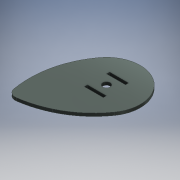
# Autodesk Inventor part: leva00
Saved by Autodesk Inventor 2016 (Build 200138000, 138)
## iProperties
Created: 2016-09-20
Part Number: leva00
Material: Madera (abedul)
Document SubType Name: Modeling
Designer: i95sa
Density: 0.55 g/cm^3
Appearance: Gris plomo - Pulido
Author: i95sa
Autodesk Inventor part; units mm, degrees
ref_plane "YZ Plane" through (0, 0, 0) normal (1, 0, 0) x (0, 1, 0)
ref_plane "XZ Plane" through (0, 0, 0) normal (0, 1, 0) x (-1, 0, 0)
ref_plane "XY Plane" through (0, 0, 0) normal (0, 0, 1) x (1, 0, 0)
sketch "Boceto1" plane through (0, 0, 0) normal (0, 0, 1) x (1, 0, 0)
  arc A0 (26.1711, 36.0215) -> (-26.1711, -36.0215) centre (0, 0) ccw
  arc A1 (-40.2753, -55.4342) -> (-52.3543, -72.0595) centre (-46.3148, -63.7469) ccw
  line L0 (-54.1029, -74.4662) -> (-62.4155, -68.4268)
  line L1 (-35.7089, 26.596) -> (-49.5634, 36.6618)
  line L2 (-49.5634, 36.6618) -> (-62.4155, -68.4268)
  line L3 (-62.4155, -68.4268) -> (-57.4262, -27.6307)
  arc A2 (-35.7089, 26.596) -> (-57.4262, -27.6307) centre (55.6688, -41.4621) ccw
  arc A3 (-57.4262, -27.6307) -> (-56.4346, -65.5259) centre (70.2836, -43.2495) ccw
  line L4 (2.0132, 2.7709) -> (26.1711, 36.0215)
  line L5 (-2.0132, -2.7709) -> (-54.1029, -74.4662)
  arc A4 (-26.1711, -36.0215) -> (26.1711, 36.0215) centre (0, 0) ccw
  arc A5 (-52.3543, -72.0595) -> (-40.2753, -55.4342) centre (-46.3148, -63.7469) ccw
  line L6 (-54.1029, -74.4662) -> (-45.7902, -80.5057)
  line L7 (36.329, -25.7426) -> (50.1834, -35.8084)
  line L8 (50.1834, -35.8084) -> (-45.7902, -80.5057)
  line L9 (-45.7902, -80.5057) -> (-8.5327, -63.154)
  arc A6 (-8.5327, -63.154) -> (36.329, -25.7426) centre (-56.6354, 40.1317) ccw
  arc A7 (-44.8796, -73.9211) -> (-8.5327, -63.154) centre (-62.8515, 53.4789) ccw
  dimension "d0" = 89.05
  dimension "d6" = 20.55
  dimension "d7" = 10.275
  dimension "d8" = 17.125
  dimension "d9" = 41.1
  constraints: 20 end point, 20 point on circle, 8 centre point, 6 symmetric about line, 5 point on line, 4 tangent, 1 collinear, 4 other
  measures "d0" diameter of A0
  measures "d6" diameter of A1
  measures "d7" distance of L0.start L0.end
  measures "d8" distance of L1.start L1.end
  measures "d9" distance of L0.end L3.end
extrude "Extrusión2" add sketch "Boceto1" along normal blind 4 contours A4 A0 | A0 L5 A1 A3 A2 | A6 A7 A5 L5 A4 | L5 A1 | A5 L5
sketch "Boceto2" plane through (0, 0, 4) normal (0, 0, 1) x (1, 0, 0)
  line L0 (0, 0) -> (0, 12.5)
  line L1 (0, 12.5) -> (-12.5, 12.5)
  line L2 (-12.5, 12.5) -> (-12.5, 16.7)
  line L3 (-12.5, 16.7) -> (12.5, 16.7)
  line L4 (12.5, 16.7) -> (12.5, 12.5)
  line L5 (12.5, 12.5) -> (0, 12.5)
  line L6 (0, 0) -> (12.5, 0)
  line L7 (0, 0) -> (0, -12.5)
  line L8 (0, -12.5) -> (-12.5, -12.5)
  line L9 (-12.5, -12.5) -> (-12.5, -16.7)
  line L10 (-12.5, -16.7) -> (12.5, -16.7)
  line L11 (12.5, -16.7) -> (12.5, -12.5)
  line L12 (12.5, -12.5) -> (0, -12.5)
  circle A0 centre (0, 0) radius 5
  dimension "d24" = 12.5
  dimension "d25" = 12.5
  dimension "d26" = 4.2
  dimension "d27" = 25
  dimension "d28" = 10
  constraints: 26 end point, 5 perpendicular, 5 symmetric about line, 3 point on line, 1 centre point, 1 coincident, 1 parallel, 1 vertical
  measures "d24" distance of L0.start L0.end
  measures "d25" distance of L0.end L1.end
  measures "d26" distance of L1.end L2.end
  measures "d27" distance of L2.end L3.end
  measures "d28" diameter of A0
extrude "Extrusión3" cut sketch "Boceto2" against normal blind 4
